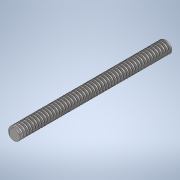
# Autodesk Inventor part: ACMET8x100mmShaft
Saved by Autodesk Inventor 2021 (Build 250183000, 183)
## iProperties
Created: 2021-03-11
Part Number: ACMET8x100mmShaft
Material: Generic
Document SubType Name: Modeling
Designer: elmar
Density: 1 g/cm^3
Appearance: Stainless - Brushed
Author: elmar
Autodesk Inventor part; units mm, degrees
ref_plane "YZ Plane" through (0, 0, 0) normal (1, 0, 0) x (0, 1, 0)
ref_plane "XZ Plane" through (0, 0, 0) normal (0, 1, 0) x (-1, 0, 0)
ref_plane "XY Plane" through (0, 0, 0) normal (0, 0, 1) x (1, 0, 0)
sketch "Sketch1" plane through (0, 0, 0) normal (0, 0, 1) x (1, 0, 0)
  circle A0 centre (0, 0) radius 4
  dimension "d0" = 8
  constraints: 1 centre point, 1 coincident
  measures "d0" diameter of A0
extrude "Extrusion1" add sketch "Sketch1" along normal blind 100
sketch "Sketch6" plane through (0, 0, 0) normal (0, 1, 0) x (-1, 0, 0)
  line L0 (0, -20) -> (0, 120) projected
  line L1 (5.6, 0) -> (-5.6, 0) projected
  line L2 (-4, -1.2679) -> (-3, -1)
  line L3 (-3, -1) -> (-3, -0.2679)
  line L4 (4, 0) -> (-4, 0) projected
  line L5 (-3, -0.2679) -> (-4, 0)
  line L6 (-4, 0) -> (-4, -1.2679)
  point P0 (0, 0)
  point P1 (-3.5, -1.134)
  point P2 (-3.5, -0.134)
  dimension "d24" = 3
  dimension "d25" = 1
  dimension "d26" = 30
  constraints: 8 end point, 2 midpoint, 1 equal length, 1 perpendicular, 1 vertical
  measures "d24" distance between parallel lines of L0 L3
  measures "d25" distance of point (-3.5, -0.134) point (-3.5, -1.134)
  measures "d26" angle of L5 L2
coil "Coil2" sketch "Sketch6" operation cut axis through (0, 0, -10) along (0, 0, 1) pitch 2 turns 51 hand right
equation "\"d12\" = 55deg"
equation "\"Sketch3_Pitch\" = 1.5"
body "Solid1"
